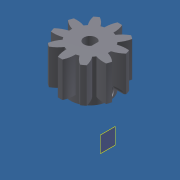
# Autodesk Inventor part: Stirnzahnrad2
Saved by Autodesk Inventor 2014 SP2 (Build 180246200, 246)
## iProperties
Created: 2014-12-12
Part Number: Stirnzahnrad2
Material: Steel
Document SubType Name: Modeling
Designer: 4ndreas
Categories: <?xml version="1.0" encoding="UTF-16"?> <MemberInstance><Categories><FamilyTemplate><FamilyTemplateParameter ValueType="xs:double" Id="1" ObjectReferenceKey="da_z" ObjectType="kUserParameterObject"/><FamilyTemplateParameter ValueType="xs:double" Id="2" ObjectReferenceKey="da_b" ObjectType="kUserParameterObject"/><FamilyTemplateParameter ValueType="xs:double" Id="3" ObjectReferenceKey="da_beta" ObjectType="kUserParameterObject"/><FamilyTemplateParameter ValueType="xs:double" Id="4" ObjectReferenceKey="da_da" ObjectType="kUserParameterObject"/><FamilyTemplateParameter ValueType="xs:double" Id="5" ObjectReferenceKey="da_aw" ObjectType="kUserParameterObject"/><FamilyTemplateParameter ValueType="xs:string" Id="6" ObjectReferenceKey="EAIAABAAAACIAQAAAAAAAIAAAAAAAAAA" ObjectType="83910656" SubObjectId="SurfaceGeometry"/></FamilyTemplate><ParamToTemplateMap><ParamToTemplate CategoryParameter="//CategoryParameter[@InternalName='046C89C9-8512-4d59-83FE-43B91F4F132A']" TemplateParameter="1"/><ParamToTemplate CategoryParameter="//CategoryParameter[@InternalName='2552DF32-E462-4b46-AEBF-C6C7768E72AC']" TemplateParameter="2"/><ParamToTemplate CategoryParameter="//CategoryParameter[@InternalName='C9EE641D-15FC-4fae-A226-E94C4372FDD7']" TemplateParameter="3"/><ParamToTemplate><ParamToTemplate CategoryParameter="//CategoryParameter[@InternalName='00B6519A-459B-49c7-AD84-2E56D39A5744']" ConstantValue="0.402671"/></ParamToTemplate><ParamToTemplate><ParamToTemplate CategoryParameter="//CategoryParameter[@InternalName='04B31F0E-C7A6-4894-AA32-9629BEFACF47']" ConstantValue="1.000000"/></ParamToTemplate><ParamToTemplate><ParamToTemplate CategoryParameter="//CategoryParameter[@InternalName='43CBEC2E-7847-49e7-A936-2F7889FCB2D9']" ConstantValue="0.250000"/></ParamToTemplate><ParamToTemplate><ParamToTemplate CategoryParameter="//CategoryParameter[@InternalName='B1EFC894-105D-4ebd-86BF-FA20ED196853']" ConstantValue="0.350000"/></ParamToTemplate><ParamToTemplate><ParamToTemplate CategoryParameter="//CategoryParameter[@InternalName='51175063-3D10-4879-93E8-6246FE8B403D']" ConstantValue="2060000000.000000"/></ParamToTemplate><ParamToTemplate><ParamToTemplate CategoryParameter="//CategoryParameter[@InternalName='A3A52E27-4454-46a9-B0BD-C932399B70AF']" ConstantValue="0.300000"/></ParamToTemplate><ParamToTemplate><ParamToTemplate CategoryParameter="//CategoryParameter[@InternalName='91B76062-C214-41d9-B1B9-14D2AB99603D']" ConstantValue="0.200000"/></ParamToTemplate><ParamToTemplate><ParamToTemplate CategoryParameter="//CategoryParameter[@InternalName='374E806E-8B8A-4dda-A9AA-1039D6500AD2']" ConstantValue="5.000000"/></ParamToTemplate><ParamToTemplate><ParamToTemplate CategoryParameter="//CategoryParameter[@InternalName='2D373A89-B862-43d6-8D0B-0CBF12AB9F6C']" ConstantValue="0.349066"/></ParamToTemplate><ParamToTemplate CategoryParameter="//CategoryParameter[@InternalName='37777632-D6A2-4fac-9D53-DB8ACD95C989']" TemplateParameter="4"/><ParamToTemplate CategoryParameter="//CategoryParameter[@InternalName='FD1017F1-B727-4f7e-9707-0F86F1FF9423']" TemplateParameter="5"/><ParamToTemplate><ParamToTemplate CategoryParameter="//CategoryParameter[@InternalName='9E1B4470-B2D3-4ff1-B813-535BB4CDF51A']" ConstantValue="3520000.000000"/></ParamToTemplate><ParamToTemplate><ParamToTemplate CategoryParameter="//CategoryParameter[@InternalName='F8452263-BFF6-458c-9FB1-07C4B99E95CD']" ConstantValue="11400000.000000"/></ParamToTemplate><ParamToTemplate><ParamToTemplate CategoryParameter="//CategoryParameter[@InternalName='3E3BB259-FD49-497f-8171-6EBC954A3479']" ConstantValue="2.000000"/></ParamToTemplate><ParamToTemplate CategoryParameter="//CategoryParameter[@InternalName='27C3BAF2-7550-4e4b-AE2C-0DB134B7D9B7']" TemplateParameter="6"/></ParamToTemplateMap><Category DisplayName="Gear" InternalName="DC85795E-93AB-48d5-8EEE-5A27447B64BD" Mnemonic="Gear"><CategoryParameter DisplayName="z" InternalName="046C89C9-8512-4d59-83FE-43B91F4F132A" Mnemonic="z"/><CategoryParameter DisplayName="b" InternalName="2552DF32-E462-4b46-AEBF-C6C7768E72AC" Mnemonic="b"/><CategoryParameter DisplayName="||b|" InternalName="C9EE641D-15FC-4fae-A226-E94C4372FDD7" Mnemonic="beta"/><CategoryParameter DisplayName="x" InternalName="00B6519A-459B-49c7-AD84-2E56D39A5744" Mnemonic="x"/><CategoryParameter DisplayName="a*" InternalName="04B31F0E-C7A6-4894-AA32-9629BEFACF47" Mnemonic="a"/><CategoryParameter DisplayName="c*" InternalName="43CBEC2E-7847-49e7-A936-2F7889FCB2D9" Mnemonic="c"/><CategoryParameter DisplayName="r|.f|*" InternalName="B1EFC894-105D-4ebd-86BF-FA20ED196853" Mnemonic="rf"/><CategoryParameter DisplayName="E" InternalName="51175063-3D10-4879-93E8-6246FE8B403D" Mnemonic="E"/><CategoryParameter DisplayName="||m|" InternalName="A3A52E27-4454-46a9-B0BD-C932399B70AF" Mnemonic="mi"/><Category DisplayName="SpurGear" InternalName="26C5A22E-A91E-4dfd-A3B3-23CCAFAE1764" Mnemonic="SpurGear"><CategoryParameter DisplayName="m" InternalName="91B76062-C214-41d9-B1B9-14D2AB99603D" Mnemonic="m"/><CategoryParameter DisplayName="P" InternalName="374E806E-8B8A-4dda-A9AA-1039D6500AD2" Mnemonic="PP"/><CategoryParameter DisplayName="||a|" InternalName="2D373A89-B862-43d6-8D0B-0CBF12AB9F6C" Mnemonic="alpha"/><CategoryParameter DisplayName="d|.a|" InternalName="37777632-D6A2-4fac-9D53-DB8ACD95C989" Mnemonic="da"/><CategoryParameter DisplayName="a|.w|" InternalName="FD1017F1-B727-4f7e-9707-0F86F1FF9423" Mnemonic="aw"/><CategoryParameter DisplayName="||s||.Flim|" InternalName="9E1B4470-B2D3-4ff1-B813-535BB4CDF51A" Mnemonic="sFlim"/><CategoryParameter DisplayName="||s||.Hlim|" InternalName="F8452263-BFF6-458c-9FB1-07C4B99E95CD" Mnemonic="sHlim"/><CategoryParameter DisplayName="Typ" InternalName="3E3BB259-FD49-497f-8171-6EBC954A3479" Mnemonic="type"/><CategoryParameter DisplayName="PitchDiameter" InternalName="27C3BAF2-7550-4e4b-AE2C-0DB134B7D9B7" Mnemonic="IDS_PITCHDIAM"/></Category></Category></Categories></MemberInstance>
Density: 1 g/cm^3
Appearance: Steel
CustomPartVersion: 1
Author: 4ndreas
Autodesk Inventor part; units mm, degrees
sketch "Sketch1" plane through (0, 0, 0) normal (0, 0, 1) x (1, 0, 0)
  circle A0 centre (0, 0) radius 12.7686
  dimension "d0" = 25.5371
  constraints: 1 centre point
  measures "d0" diameter of A0
extrude "Extrusion1" add sketch "Sketch1" along normal blind 15
ref_plane "Work Plane2" through (0, 0, 7.5) normal (0, 0, 1) x (1, 0, 0)
sketch "Sketch2" plane through (0, 0, 0) normal (0, 0, -1) x (-1, 0, 0)
  circle A0 centre (0, 0) radius 12.7686 projected
  circle A1 centre (0, 0) radius 10.1325
  dimension "d3" = 20.265
  constraints: 1 centre point, 1 coincident
  measures "d3" diameter of A1
surface extrude "Flankendurchmesser" sketch "Sketch2" against normal through all shown no curves A1
ref_plane "Work Plane8" through (0, 0, 0) normal (0.9510565, 0.309017, 0) x (0, 0, 1)
ref_plane "Work Plane9" through (0, 0, 0) normal (1, 0, 0) x (0, 1, 0)
spur gear teeth "Stirnzahnrad" teeth 10 pitch diameter 20 tip diameter 25.5371 root diameter 16.6107 face width 15 start plane through (0, 0, 0) normal (0, 0, -1) x (-1, 0, 0)
sketch "Skizze3" plane through (0, 0, 0) normal (0, 0, -1) x (-1, 0, 0)
  arc A0 (-6.6716, 10.887) -> (-8.2925, 9.7093) centre (0, 0) ccw
  circle A1 centre (0, 0) radius 8.3053
  arc A2 (6.3154, 5.3939) -> (8.2925, 9.7093) centre (-2.2863, 11.9453) ccw projected
  arc A3 (8.2925, 9.7093) -> (6.6716, 10.887) centre (0, 0) ccw projected
  arc A4 (6.6716, 10.887) -> (3.1783, 7.6731) centre (12.0672, 1.5169) ccw projected
  arc A5 (3.1783, 7.6731) -> (1.9388, 8.0759) centre (0, 0) ccw projected
  arc A6 (1.9388, 8.0759) -> (1.0018, 12.7292) centre (-8.871, 8.3201) ccw projected
  arc A7 (1.0018, 12.7292) -> (-1.0018, 12.7292) centre (0, 0) ccw projected
  arc A8 (-1.0018, 12.7292) -> (-1.9388, 8.0759) centre (8.871, 8.3201) ccw projected
  arc A9 (-1.9388, 8.0759) -> (-3.1783, 7.6731) centre (0, 0) ccw projected
  arc A10 (-3.1783, 7.6731) -> (-6.6716, 10.887) centre (-12.0672, 1.5169) ccw projected
  arc A11 (-6.6716, 10.887) -> (-8.2925, 9.7093) centre (0, 0) ccw projected
  arc A12 (-8.2925, 9.7093) -> (-6.3154, 5.3939) centre (2.2863, 11.9453) ccw projected
  arc A13 (-6.3154, 5.3939) -> (-7.0815, 4.3395) centre (0, 0) ccw projected
  arc A14 (-7.0815, 4.3395) -> (-11.7966, 4.8863) centre (-10.6542, -5.8657) ccw projected
  arc A15 (-11.7966, 4.8863) -> (-12.4158, 2.9808) centre (0, 0) ccw projected
  arc A16 (-12.4158, 2.9808) -> (-8.2797, 0.6516) centre (-5.1716, 11.0078) ccw projected
  arc A17 (-8.2797, 0.6516) -> (-8.2797, -0.6516) centre (0, 0) ccw projected
  arc A18 (-8.2797, -0.6516) -> (-12.4158, -2.9808) centre (-5.1716, -11.0078) ccw projected
  arc A19 (-12.4158, -2.9808) -> (-11.7966, -4.8863) centre (0, 0) ccw projected
  arc A20 (-11.7966, -4.8863) -> (-7.0815, -4.3395) centre (-10.6542, 5.8657) ccw projected
  arc A21 (-7.0815, -4.3395) -> (-6.3154, -5.3939) centre (0, 0) ccw projected
  arc A22 (-6.3154, -5.3939) -> (-8.2925, -9.7093) centre (2.2863, -11.9453) ccw projected
  arc A23 (-8.2925, -9.7093) -> (-6.6716, -10.887) centre (0, 0) ccw projected
  arc A24 (-6.6716, -10.887) -> (-3.1783, -7.6731) centre (-12.0672, -1.5169) ccw projected
  arc A25 (-3.1783, -7.6731) -> (-1.9388, -8.0759) centre (0, 0) ccw projected
  arc A26 (-1.9388, -8.0759) -> (-1.0018, -12.7292) centre (8.871, -8.3201) ccw projected
  arc A27 (-1.0018, -12.7292) -> (1.0018, -12.7292) centre (0, 0) ccw projected
  arc A28 (1.0018, -12.7292) -> (1.9388, -8.0759) centre (-8.871, -8.3201) ccw projected
  arc A29 (1.9388, -8.0759) -> (3.1783, -7.6731) centre (0, 0) ccw projected
  arc A30 (3.1783, -7.6731) -> (6.6716, -10.887) centre (12.0672, -1.5169) ccw projected
  arc A31 (6.6716, -10.887) -> (8.2925, -9.7093) centre (0, 0) ccw projected
  arc A32 (8.2925, -9.7093) -> (6.3154, -5.3939) centre (-2.2863, -11.9453) ccw projected
  arc A33 (6.3154, -5.3939) -> (7.0815, -4.3395) centre (0, 0) ccw projected
  arc A34 (7.0815, -4.3395) -> (11.7966, -4.8863) centre (10.6542, 5.8657) ccw projected
  arc A35 (11.7966, -4.8863) -> (12.4158, -2.9808) centre (0, 0) ccw projected
  arc A36 (12.4158, -2.9808) -> (8.2797, -0.6516) centre (5.1716, -11.0078) ccw projected
  arc A37 (8.2797, -0.6516) -> (8.2797, 0.6516) centre (0, 0) ccw projected
  arc A38 (8.2797, 0.6516) -> (12.4158, 2.9808) centre (5.1716, 11.0078) ccw projected
  arc A39 (12.4158, 2.9808) -> (11.7966, 4.8863) centre (0, 0) ccw projected
  arc A40 (11.7966, 4.8863) -> (7.0815, 4.3395) centre (10.6542, -5.8657) ccw projected
  arc A41 (7.0815, 4.3395) -> (6.3154, 5.3939) centre (0, 0) ccw projected
  constraints: 2 centre point, 2 point on circle, 1 coincident
extrude "Extrusion2" add sketch "Skizze3" along normal blind 3 contours A1
sketch "Skizze4" plane through (0, 0, 0) normal (1, 0, 0) x (0, 1, 0)
  circle A0 centre (0, 0) radius 1.6
  dimension "d51" = 3.2
  constraints: 1 centre point, 1 coincident
  measures "d51" diameter of A0
hole "Bohrung1" at (0, 0, -3) direction (0, 0, 1) diameter 5.2 end through all
sketch "Skizze5" plane through (0, 0, -3) normal (0, 0, -1) x (-1, 0, 0)
  circle A0 centre (0, 0) radius 2.6 projected
  circle A1 centre (0, 0) radius 8.3053 projected
  line L0 (-2.1298, 1.4913) -> (-2.1298, -1.4913)
  line L1 (0, 0) -> (0, 4.533) construction
  line L2 (0, 4.533) -> (-2.1298, 1.4913) construction
  dimension "d65" = 35
  constraints: 6 end point, 2 point on circle, 1 parallel, 1 tangent, 1 vertical
  measures "d65" angle of L1 L2
extrude "Extrusion4" add sketch "Skizze5" against normal up to surface (18 mm away) contours L0 A0 picked at (-2.229, -0.3106)
extrude "Extrusion3" cut sketch "Skizze4" along normal through all
ref_plane "Arbeitsebene11" through (4.6298, -1.4913, -3) normal (-1, 0, 0) x (0, 0, 1)
sketch "Skizze6" plane through (4.6298, -1.4913, -3) normal (-1, 0, 0) x (0, 0, 1)
  arc A0 (2.4203, 2.9826) -> (2.4203, 0) centre (3, 1.4913) ccw projected
  arc A1 (3.5797, 0) -> (3.5797, 2.9826) centre (3, 1.4913) ccw projected
  line L0 (6.2909, 1.4913) -> (4.6454, -1.3587)
  line L1 (4.6454, -1.3587) -> (1.3546, -1.3587)
  line L2 (1.3546, -1.3587) -> (-0.2909, 1.4913)
  line L3 (-0.2909, 1.4913) -> (1.3546, 4.3413)
  line L4 (1.3546, 4.3413) -> (4.6454, 4.3413)
  line L5 (4.6454, 4.3413) -> (6.2909, 1.4913)
  line L6 (1.3546, -1.3587) -> (-2, -1.3587)
  line L7 (-2, -1.3587) -> (-2, 4.3413)
  line L8 (-2, 4.3413) -> (1.3546, 4.3413)
  line L9 (1.3546, 4.3413) -> (1.3546, -1.3587)
  line L10 (0, 9.7966) -> (0, -6.814) projected
  point P0 (3, 1.4913)
  dimension "d69" = 5.7
  dimension "d70" = 2
  constraints: 20 end point, 2 horizontal, 2 horizontal alignment, 2 parallel, 2 vertical alignment, 1 coincident, 1 collinear, 1 perpendicular, 15 other
  measures "d69" distance between parallel lines of L4 L1
  measures "d70" distance between parallel lines of L10 L7
extrude "Extrusion5" cut sketch "Skizze6" along normal mid plane 3
ref_plane "Arbeitsebene12" through (7.6298, -1.4913, -3) normal (-1, 0, 0) x (0, 0, 1)
sketch "Skizze7" plane through (7.6298, -1.4913, -3) normal (-1, 0, 0) x (0, 0, 1)
  circle A0 centre (3, 1.4913) radius 2.5
  dimension "d74" = 5
  constraints: 1 centre point, 1 coincident
  measures "d74" diameter of A0
extrude "Extrusion6" cut sketch "Skizze7" against normal through all
chamfer "Fase1" distance 0.5 angle 45 1 edges at (7.6298, -1.6, 0)
equation "\"d0\" = da_da"
equation "\"d1\" = da_b"
equation "\"d3\" = da_dw"
equation "\"d16\" = da_aw"
equation "\"d43\" = da_aw"
equation "\"d46\" = da_aw"
equation "\"da_da\" = 25.537132"
equation "\"da_b\" = 15"
equation "\"da_dw\" = 20.265023"
equation "\"da_aw\" = 58.768566"
body "Solid1"
body "Srf1"
